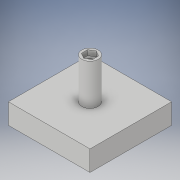
# Autodesk Inventor part: YMount_Belt
Saved by Autodesk Inventor 2018 (Build 220112000, 112)
## iProperties
Created: 2020-03-14
Part Number: YMount_Belt
Material: Generic
Document SubType Name: Modeling
Designer: natha
Density: 1 g/cm^3
Appearance: Default
Author: natha
Autodesk Inventor part; units mm, degrees
ref_plane "YZ Plane" through (0, 0, 0) normal (1, 0, 0) x (0, 1, 0)
ref_plane "XZ Plane" through (0, 0, 0) normal (0, 1, 0) x (-1, 0, 0)
ref_plane "XY Plane" through (0, 0, 0) normal (0, 0, 1) x (1, 0, 0)
sketch "Sketch1" plane through (0, 0, 0) normal (0, 1, 0) x (-1, 0, 0)
  line L0 (0, 0) -> (40, 0)
  line L1 (40, 0) -> (40, -40)
  line L2 (40, -40) -> (0, -40)
  line L3 (0, -40) -> (0, 0)
  dimension "d0" = 40
  dimension "d1" = 40
  constraints: 8 end point, 2 parallel, 1 horizontal, 1 perpendicular
  measures "d0" distance of L1.end L2.end
  measures "d1" distance of L0.end L1.end
extrude "Extrusion1" add sketch "Sketch1" along normal blind 10
sketch "Sketch2" plane through (0, 10, 0) normal (0, 1, 0) x (1, 0, 0)
  circle A0 centre (-20, 20) radius 4
  point P0 (0, 0)
  dimension "d4" = 8
  constraints: 1 centre point
  measures "d4" diameter of A0
extrude "Extrusion2" add sketch "Sketch2" along normal blind 20
sketch "Sketch3" plane through (-20, 30, -20) normal (0, 1, 0) x (1, 0, 0)
  line L0 (2.6327, 1.6155) -> (2.7154, -1.4722)
  line L1 (2.7154, -1.4722) -> (0.0827, -3.0877)
  line L2 (0.0827, -3.0877) -> (-2.6327, -1.6155)
  line L3 (-2.6327, -1.6155) -> (-2.7154, 1.4722)
  line L4 (-2.7154, 1.4722) -> (-0.0827, 3.0877)
  line L5 (-0.0827, 3.0877) -> (2.6327, 1.6155)
  point P0 (20, -20)
  point P1 (0, 0)
  dimension "d7" = 5.35
  constraints: 12 end point, 13 other
  measures "d7" distance between parallel lines of L3 L0
extrude "Extrusion3" cut sketch "Sketch3" against normal blind 2.5
sketch "Sketch4" plane through (-20, 27.5, -20) normal (0, 1, 0) x (1, 0, 0)
  circle A0 centre (0, 0) radius 1.375
  point P0 (20, -20)
  dimension "d10" = 2.75
  constraints: 1 centre point
  measures "d10" diameter of A0
extrude "Extrusion4" cut sketch "Sketch4" against normal blind 2.5
body "Solid1"
